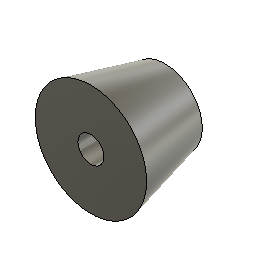
3D Printed Foot 3mm (Autodesk Fusion 360 design; units mm, degrees)
Autodesk Fusion 360 part; units mm, degrees
sketch "Sketch1" plane through (0, 0, 0) normal (0, 1, 0) x (1, 0, 0)
  line L0 (-2, 0) -> (-4.5, -10)
  line L1 (-4.5, -10) -> (3, -10)
  line L2 (3, -10) -> (3, -4)
  line L3 (3, -4) -> (0, -4)
  line L4 (0, -4) -> (0, 0)
  line L5 (-2, 0) -> (0, 0)
  line L6 (3, -10) -> (3, 0.0112) construction
  line L7 (1.25, -4) -> (1.25, -10)
  dimension "d1" = 3
  dimension "d2" = 6
  dimension "d3" = 4
  dimension "d4" = 2
  dimension "d5" = 7.5
  dimension "d8" = 1.75
  measures "d3" distance of L4.end
  measures "d4" distance of L4.end
revolve "Revolve1" add sketch "Sketch1" angle 360 about axis through (3, 0, 10) along (0, 0, -1) contours L0 L1 L3 L4 L5 L7
fillet "Fillet1" [suppressed]
named bodies: "3mm foot"
